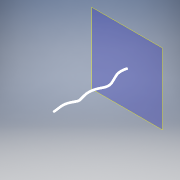
# Autodesk Inventor part: spark
Saved by Autodesk Inventor 2017 (Build 210142000, 142)
## iProperties
Part Number: spark
Material: Generisch
Document SubType Name: Modeling
Designer: David Merges
Density: 1 g/cm^3
Appearance: Vorgabe
Author: David Merges
Autodesk Inventor part; units mm, degrees
ref_plane "YZ Plane" through (0, 0, 0) normal (1, 0, 0) x (0, 1, 0)
ref_plane "XY Plane" through (0, 0, 0) normal (0, 0, 1) x (1, 0, 0)
sketch "Skizze1" plane through (0, 0, 0) normal (0, 0, 1) x (1, 0, 0)
  line L0 (0.1011, 1.5184) -> (0.2351, 1.2374)
  line L1 (0.231, 0.7986) -> (0.1694, 0.6754)
  line L2 (0.0977, -0.0297) -> (0.18, -0.3379)
  line L3 (0.1656, -0.4789) -> (0.0654, -0.6794)
  line L4 (-0.0123, -1.1404) -> (0.0379, -1.5263)
  arc A0 (0.231, 0.7986) -> (0.2351, 1.2374) centre (-0.2162, 1.0222) ccw
  arc A1 (0.1694, 0.6754) -> (0.0977, -0.0297) centre (1.0639, 0.2282) ccw
  arc A2 (0.1656, -0.4789) -> (0.18, -0.3379) centre (-0.0133, -0.3895) ccw
  line L5 (-1.5, 2.5) -> (1.5, 2.5) projected
  line L6 (1.5, -2.5) -> (-1.5, -2.5) projected
  line L7 (1.5, 2.5) -> (1.5, -2.5) projected
  line L8 (-1.5, 2.5) -> (1.5, 2.5) projected
  line L9 (1.5, -2.5) -> (-1.5, -2.5) projected
  line L10 (1.5, 2.5) -> (1.5, -2.5) projected
  arc A3 (0.0654, -0.6794) -> (-0.0123, -1.1404) centre (0.781, -1.0371) ccw
  line L11 (0.0357, 1.6556) -> (0.1011, 1.5184)
  arc A4 (0, 2.2563) -> (0.0357, 1.6556) centre (0.7578, 1.9999) ccw
  line L12 (-1.5, -2.5) -> (-1.5, 2.5) projected
  line L13 (-1.5, -2.5) -> (-1.5, 2.5) projected
  point P0 (0, 0)
  dimension "d0" = 0.5
  dimension "d1" = 1
  dimension "d2" = 0.2
  dimension "d3" = 0.8
  dimension "d4" = 0.8
  constraints: 12 end point, 10 point on circle, 9 tangent, 5 centre point, 1 coincident, 1 collinear, 1 parallel
  measures "d0" radius of A0
  measures "d1" radius of A1
  measures "d2" radius of A2
  measures "d3" radius of A3
  measures "d4" radius of A4
ref_plane "Arbeitsebene1" through (0, 2.2563, 0) normal (0, 1, 0) x (-1, 0, 0)
sketch "Skizze2" plane through (0, 2.2563, 0) normal (0, 1, 0) x (-1, 0, 0)
  circle A0 centre (0, 0) radius 0.05
  point P0 (0, 0)
  dimension "d5" = 0.1
  constraints: 1 centre point, 1 coincident
  measures "d5" diameter of A0
sweep "Sweeping1" add profiles "Skizze2" path "Skizze1" path curves A4 L11 L0 A0 L1 A1 L2 A2 L3 A3 L4
